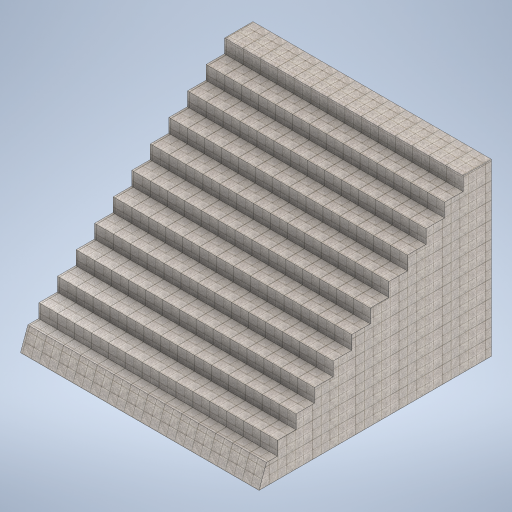
# Autodesk Inventor part: side_stair
Saved by Autodesk Inventor 2024.2 (Build 282272000, 272)
## iProperties
Created: 2024-05-25
Part Number: side_stair
Material: Generic
Document SubType Name: Modeling
Designer: LOSTER_1
Density: 1 g/cm^3
Appearance: Default
Author: LOSTER_1
Autodesk Inventor part; units mm, degrees
ref_plane "YZ Plane" through (0, 0, 0) normal (1, 0, 0) x (0, 1, 0)
ref_plane "XZ Plane" through (0, 0, 0) normal (0, 1, 0) x (-1, 0, 0)
ref_plane "XY Plane" through (0, 0, 0) normal (0, 0, 1) x (1, 0, 0)
sketch "Sketch1" plane through (0, 0, 0) normal (0, 1, 0) x (-1, 0, 0)
  line L0 (1400, 1000) -> (-1400, 1000)
  line L1 (-1400, 1000) -> (-1400, -1000)
  line L2 (-1400, -1000) -> (1400, -1000)
  line L3 (1400, -1000) -> (1400, 1000)
  line L4 (1400, 1000) -> (-1400, -1000) construction
  line L5 (-1400, 1000) -> (1400, -1000) construction
  point P0 (0, 0)
  dimension "d0" = 2800
  dimension "d1" = 2000
  constraints: 12 end point, 2 midpoint, 2 parallel, 1 horizontal, 1 perpendicular
  measures "d0" distance of L2.end L1.end
  measures "d1" distance of L1.end L0.end
extrude "Extrusion1" add sketch "Sketch1" along normal blind 2000
sketch "Sketch2" plane through (1400, 0, 1000) normal (1, 0, 0) x (0, 0, -1)
  line L0 (0, 2000) -> (2000, 2000) projected
  line L1 (0, 0) -> (2000, 0) projected
  line L2 (0, 2000) -> (0, 0)
  line L3 (0, 0) -> (-727.9405, 0)
  line L4 (0, 2000) -> (-727.9405, 0)
  line L5 (0, 2000) -> (2128.3555, 2000) construction
  point P0 (1000, 0)
  dimension "d4" = 110
  constraints: 8 end point, 2 perpendicular, 1 equal length, 1 horizontal
  measures "d4" angle of L4 L5
extrude "Extrusion2" add sketch "Sketch2" against normal blind 2800
sketch "Sketch3" plane through (1400, 0, -1000) normal (1, 0, 0) x (0, 0, -1)
  line L0 (-2.1545, -0.4275) -> (-2.1545, 1999.5725)
  line L1 (-2.1545, -0.4275) -> (-2.1545, 159.5725)
  line L2 (-2.1545, 159.5725) -> (-2.1545, 319.5725)
  line L3 (-2.1545, 319.5725) -> (-2.1545, 479.5725)
  line L4 (-2.1545, 479.5725) -> (-2.1545, 639.5725)
  line L5 (-2.1545, 639.5725) -> (-2.1545, 799.5725)
  line L6 (-2.1545, 799.5725) -> (-2.1545, 959.5725)
  line L7 (-2.1545, 959.5725) -> (-2.1545, 1119.5725)
  line L8 (-2.1545, 1119.5725) -> (-2.1545, 1279.5725)
  line L9 (-2.1545, 1279.5725) -> (-2.1545, 1439.5725)
  line L10 (-2.1545, 1439.5725) -> (-2.1545, 1599.5725)
  line L11 (-2.1545, 1599.5725) -> (-2.1545, 1759.5725)
  line L12 (-2.1545, 1759.5725) -> (-2.1545, 1919.5725)
  line L13 (-2.1545, 1919.5725) -> (-2.1545, 1999.9008)
  line L14 (-2.1545, -0.4275) -> (-2730.0949, -0.4275)
  line L15 (-2730.0949, -0.4275) -> (-2512.0949, -0.4275)
  line L16 (-2512.0949, -0.4275) -> (-2294.0949, -0.4275)
  line L17 (-2294.0949, -0.4275) -> (-2076.0949, -0.4275)
  line L18 (-2076.0949, -0.4275) -> (-1858.0949, -0.4275)
  line L19 (-1858.0949, -0.4275) -> (-1640.0949, -0.4275)
  line L20 (-1640.0949, -0.4275) -> (-1422.0949, -0.4275)
  line L21 (-1422.0949, -0.4275) -> (-1204.0949, -0.4275)
  line L22 (-1204.0949, -0.4275) -> (-986.0949, -0.4275)
  line L23 (-986.0949, -0.4275) -> (-768.0949, -0.4275)
  line L24 (-768.0949, -0.4275) -> (-550.0949, -0.4275)
  line L25 (-550.0949, -0.4275) -> (-332.0949, -0.4275)
  line L26 (-332.0949, -0.4275) -> (-114.0949, -0.4275)
  line L27 (-114.0949, -0.4275) -> (-2.1545, -0.4275)
  line L28 (-2730.0949, -0.4275) -> (-2642.7421, 239.5725)
  line L29 (-2730.0949, -0.4275) -> (-2002.1545, 1999.5725)
  line L30 (-2642.7421, 239.5725) -> (-2512.0949, 239.5725)
  line L31 (-2512.0949, 239.5725) -> (-2512.0949, 399.5725)
  line L32 (-2512.0949, 399.5725) -> (-2294.0949, 399.5725)
  line L33 (-2294.0949, 399.5725) -> (-2294.0949, 559.5725)
  line L34 (-2294.0949, 559.5725) -> (-2076.0949, 559.5725)
  line L35 (-2076.0949, 559.5725) -> (-2076.0949, 719.5725)
  line L36 (-2076.0949, 719.5725) -> (-1858.0949, 719.5725)
  line L37 (-1858.0949, 719.5725) -> (-1858.0949, 879.5725)
  line L38 (-1858.0949, 879.5725) -> (-1640.0949, 879.5725)
  line L39 (-1640.0949, 879.5725) -> (-1640.0949, 1039.5725)
  line L40 (-1640.0949, 1039.5725) -> (-1422.0949, 1039.5725)
  line L41 (-1422.0949, 1039.5725) -> (-1422.0949, 1199.5725)
  line L42 (-1422.0949, 1199.5725) -> (-1204.0949, 1199.5725)
  line L43 (-1204.0949, 1199.5725) -> (-1204.0949, 1359.5725)
  line L44 (-1204.0949, 1359.5725) -> (-986.0949, 1359.5725)
  line L45 (-986.0949, 1359.5725) -> (-986.0949, 1519.5725)
  line L46 (-986.0949, 1519.5725) -> (-768.0949, 1519.5725)
  line L47 (-768.0949, 1519.5725) -> (-768.0949, 1679.5725)
  line L48 (-768.0949, 1679.5725) -> (-550.0949, 1679.5725)
  line L49 (-550.0949, 1679.5725) -> (-550.0949, 1839.5725)
  line L50 (-550.0949, 1839.5725) -> (-332.0949, 1839.5725)
  line L51 (-332.0949, 1839.5725) -> (-332.0949, 1999.5725)
  line L52 (-332.0949, 1999.5725) -> (-2002.1545, 1999.5725)
  line L53 (-2002.1545, 1999.5725) -> (-2642.7421, 239.5725)
  line L54 (-2727.9405, 0) -> (0, 0) projected
  line L55 (-332.0949, 1999.5725) -> (-332.0949, 2182.2078)
  line L56 (-332.0949, 2182.2078) -> (-3155.7019, 2182.2078)
  line L57 (-3155.7019, 2182.2078) -> (-3155.7019, 0)
  line L58 (-3155.7019, 0) -> (-2727.9405, 0)
  point P0 (-1000, 0)
  point P1 (-1002.1545, -0.4275)
  point P2 (-2729.9393, 0)
  dimension "d7" = 160
  dimension "d8" = 160
  dimension "d9" = 160
  dimension "d10" = 160
  dimension "d11" = 160
  dimension "d12" = 160
  dimension "d13" = 160
  dimension "d14" = 160
  dimension "d15" = 160
  dimension "d16" = 160
  dimension "d17" = 160
  dimension "d18" = 160
  dimension "d19" = 218
  dimension "d20" = 218
  dimension "d21" = 218
  dimension "d22" = 218
  dimension "d23" = 218
  dimension "d24" = 218
  dimension "d25" = 218
  dimension "d26" = 218
  dimension "d27" = 218
  dimension "d28" = 218
  dimension "d29" = 218
  dimension "d30" = 218
  constraints: 112 end point, 24 perpendicular, 13 coincident, 4 point on line, 2 horizontal, 1 collinear, 1 vertical, 28 other
  measures "d7" distance of L1.start L1.end
  measures "d8" distance of L1.end L2.end
  measures "d9" distance of L2.end L3.end
  measures "d10" distance of L3.end L4.end
  measures "d11" distance of L4.end L5.end
  measures "d12" distance of L5.end L6.end
  measures "d13" distance of L6.end L7.end
  measures "d14" distance of L7.end L8.end
  measures "d15" distance of L8.end L9.end
  measures "d16" distance of L9.end L10.end
  measures "d17" distance of L10.end L11.end
  measures "d18" distance of L11.end L12.end
  measures "d19" distance of L15.start L15.end
  measures "d20" distance of L15.end L16.end
  measures "d21" distance of L16.end L17.end
  measures "d22" distance of L17.end L18.end
  measures "d23" distance of L18.end L19.end
  measures "d24" distance of L19.end L20.end
  measures "d25" distance of L20.end L21.end
  measures "d26" distance of L21.end L22.end
  measures "d27" distance of L22.end L23.end
  measures "d28" distance of L23.end L24.end
  measures "d29" distance of L24.end L25.end
  measures "d30" distance of L25.end L26.end
extrude "Extrusion3" cut sketch "Sketch3" against normal blind 2800 contours L58 L57 L56 L55 L52 L29 L28 | L29 L52 L51 L50 L49 L48 L47 L46 L45 L44 L43 L42 L41 L40 L39 L38 L37 L36 L35 L34 L33 L32 L31 L30
body "Solid1"
